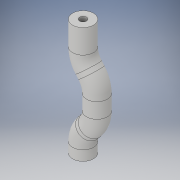
# Autodesk Inventor part: BottomTopPlateSpacer
Saved by Autodesk Inventor 2017 (Build 210142000, 142)
## iProperties
Created: 2017-09-15
Part Number: BottomTopPlateSpacer
Material: Generic
Document SubType Name: Modeling
Designer: Axel
Density: 1 g/cm^3
Appearance: Default
Author: Axel
Autodesk Inventor part; units mm, degrees
ref_plane "YZ Plane" through (0, 0, 0) normal (1, 0, 0) x (0, 1, 0)
ref_plane "XZ Plane" through (0, 0, 0) normal (0, 1, 0) x (-1, 0, 0)
ref_plane "XY Plane" through (0, 0, 0) normal (0, 0, 1) x (1, 0, 0)
sketch "Sketch1" plane through (0, 0, 0) normal (0, 1, 0) x (-1, 0, 0)
  circle A0 centre (0, 0) radius 1.5
  circle A1 centre (0, 0) radius 4.5
  dimension "d0" = 3
  dimension "d1" = 9
  constraints: 2 centre point, 2 coincident
  measures "d0" diameter of A0
  measures "d1" diameter of A1
sketch "Sketch2" plane through (0, 0, 0) normal (0, 0, 1) x (1, 0, 0)
  line L0 (0, 0) -> (0, 4.3008)
  line L1 (2.4074, 10.8087) -> (3.5926, 12.1913)
  line L2 (6, 18.6992) -> (6, 25.3008)
  line L3 (3.5926, 31.8087) -> (2.4074, 33.1913)
  line L4 (0, 39.6992) -> (0, 50)
  line L5 (6, 22) -> (-6.3181, 22) construction
  arc A0 (2.4074, 10.8087) -> (0, 4.3008) centre (10, 4.3008) ccw
  arc A1 (3.5926, 12.1913) -> (6, 18.6992) centre (-4, 18.6992) ccw
  arc A2 (6, 25.3008) -> (3.5926, 31.8087) centre (-4, 25.3008) ccw
  arc A3 (0, 39.6992) -> (2.4074, 33.1913) centre (10, 39.6992) ccw
  point P0 (0, 8)
  point P1 (6, 15)
  point P2 (6, 29)
  point P3 (0, 36)
  dimension "d4" = 8
  dimension "d5" = 50
  dimension "d6" = 7
  dimension "d7" = 7
  dimension "d8" = 14
  dimension "d9" = 22
  dimension "d10" = 6
  dimension "d11" = 10
  constraints: 12 end point, 10 point on line, 8 point on circle, 8 tangent, 4 centre point, 3 equal radius, 1 horizontal, 1 midpoint, 1 parallel, 1 vertical
  measures "d4" distance of L0.start point (0, 8)
  measures "d5" distance of L0.start L4.end
  measures "d6" vertical distance of point (6, 15) point (0, 8)
  measures "d7" vertical distance of point (0, 36) point (6, 29)
  measures "d8" distance of point (6, 15) point (6, 29)
  measures "d9" distance from line of L0.start L5
  measures "d10" horizontal distance of point (0, 8) point (6, 15)
  measures "d11" radius of A0
sweep "Sweep1" add profiles "Sketch1" path "Sketch2"
body "Solid2"
